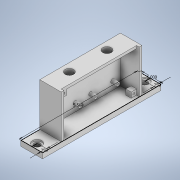
# Autodesk Inventor part: DualSensorReadout
Saved by Autodesk Inventor 2020 (Build 240168000, 168)
## iProperties
Created: 2024-01-28
Part Number: DualSensorReadout
Material: Generic
Document SubType Name: Modeling
Designer: Beaucage
Density: 1 g/cm^3
Appearance: Default
Author: Beaucage
Autodesk Inventor part; units mm, degrees
ref_plane "YZ Plane" through (0, 0, 0) normal (1, 0, 0) x (0, 1, 0)
ref_plane "XZ Plane" through (0, 0, 0) normal (0, 1, 0) x (-1, 0, 0)
ref_plane "XY Plane" through (0, 0, 0) normal (0, 0, 1) x (1, 0, 0)
sketch "Sketch1" plane through (0, 0, 0) normal (0, 1, 0) x (-1, 0, 0)
  line L0 (0, 0) -> (25.4, 0)
  line L1 (25.4, 0) -> (25.4, -139.7)
  line L2 (25.4, -139.7) -> (0, -139.7)
  line L3 (0, -139.7) -> (0, 0)
  line L4 (12.7, 0) -> (12.7, -6.35)
  line L5 (12.7, -139.7) -> (12.7, -133.35)
  dimension "d0" = 25.4
  dimension "d1" = 139.7
  dimension "d2" = 6.35
  dimension "d3" = 6.35
  constraints: 12 end point, 2 midpoint, 2 parallel, 2 vertical, 1 horizontal, 1 perpendicular
  measures "d0" distance of L1.end L2.end
  measures "d1" distance of L0.end L1.end
  measures "d2" distance of L4.start L4.end
  measures "d3" distance of L5.start L5.end
extrude "Extrusion1" add sketch "Sketch1" against normal blind 6.35
hole "Hole1" at (-12.7, 0, -6.35) at (-12.7, 0, -133.35) direction (0, -1, 0) diameter 7.1374 depth 7.9375 counterbore diameter 11.1252 counterbore depth 1.5875 clearance for "Socket Head Cap Screw" size "1/4" standard "Ansi Unified Screw Threads"
sketch "Sketch2" plane through (0, 0, 0) normal (0, 1, 0) x (1, 0, 0)
  line L0 (-25.4, 0) -> (-25.4, 139.7) projected
  line L1 (-25.4, 0) -> (-25.4, 25.4)
  line L2 (-25.4, 25.4) -> (-22.225, 25.4)
  line L3 (-22.225, 25.4) -> (-22.225, 114.3)
  line L4 (-22.225, 114.3) -> (-25.4, 114.3)
  line L5 (-25.4, 114.3) -> (-25.4, 25.4)
  line L6 (-25.4, 25.4) -> (0, 25.4)
  line L7 (0, 25.4) -> (0, 22.225)
  line L8 (0, 22.225) -> (-25.4, 22.225)
  line L9 (-25.4, 22.225) -> (-25.4, 25.4)
  line L10 (-25.4, 114.3) -> (0, 114.3)
  line L11 (0, 114.3) -> (0, 117.475)
  line L12 (0, 117.475) -> (-25.4, 117.475)
  line L13 (-25.4, 117.475) -> (-25.4, 114.3)
  point P0 (0, 0)
  dimension "d13" = 25.4
  dimension "d14" = 3.175
  dimension "d15" = 88.9
  dimension "d16" = 25.4
  dimension "d17" = 3.175
  dimension "d18" = 25.4
  dimension "d19" = 3.175
  constraints: 26 end point, 6 parallel, 3 horizontal, 3 perpendicular, 1 point on line
  measures "d13" distance of L0.start L1.end
  measures "d14" distance of L4.end L3.end
  measures "d15" distance of L3.end L2.end
  measures "d16" distance of L7.end L8.end
  measures "d17" distance of L6.end L7.end
  measures "d18" distance of L12.end L11.end
  measures "d19" distance of L11.end L10.end
extrude "Extrusion2" add sketch "Sketch2" along normal blind 50.8
sketch "Sketch3" plane through (-22.225, 0, -25.4) normal (1, 0, 0) x (0, 0, -1)
  line L0 (88.9, 0) -> (88.9, 50.8) projected
  line L1 (88.9, 50.8) -> (0, 50.8)
  line L2 (0, 50.8) -> (0, 47.625)
  line L3 (0, 47.625) -> (88.9, 47.625)
  line L4 (88.9, 47.625) -> (88.9, 50.8)
  point P0 (-25.4, 0)
  dimension "d22" = 88.9
  dimension "d23" = 3.175
  constraints: 8 end point, 2 parallel, 1 horizontal, 1 perpendicular
  measures "d22" distance of L3.end L2.end
  measures "d23" distance of L2.end L1.end
extrude "Extrusion3" add sketch "Sketch3" along normal blind 19.05
sketch "Sketch4" plane through (-22.225, 0, -25.4) normal (1, 0, 0) x (0, 0, -1)
  line L0 (88.9, 47.625) -> (0, 47.625) projected
  line L1 (44.45, 47.625) -> (44.45, 23.8125)
  line L2 (44.45, 23.8125) -> (66.675, 23.8125)
  line L3 (66.675, 23.8125) -> (22.225, 23.8125)
  line L4 (9.2075, 9.525) -> (35.2425, 9.525)
  line L5 (35.2425, 9.525) -> (35.2425, 38.1)
  line L6 (35.2425, 38.1) -> (9.2075, 38.1)
  line L7 (9.2075, 38.1) -> (9.2075, 9.525)
  line L8 (9.2075, 9.525) -> (35.2425, 38.1) construction
  line L9 (35.2425, 9.525) -> (9.2075, 38.1) construction
  line L10 (53.6575, 9.525) -> (79.6925, 9.525)
  line L11 (79.6925, 9.525) -> (79.6925, 38.1)
  line L12 (79.6925, 38.1) -> (53.6575, 38.1)
  line L13 (53.6575, 38.1) -> (53.6575, 9.525)
  line L14 (53.6575, 9.525) -> (79.6925, 38.1) construction
  line L15 (79.6925, 9.525) -> (53.6575, 38.1) construction
  circle A0 centre (9.2075, 38.1) radius 2.2225
  circle A1 centre (35.2425, 38.1) radius 2.2225
  circle A2 centre (9.2075, 9.525) radius 2.2225
  circle A3 centre (35.2425, 9.525) radius 2.2225
  circle A4 centre (53.6575, 9.525) radius 2.2225
  circle A5 centre (79.6925, 9.525) radius 2.2225
  circle A6 centre (79.6925, 38.1) radius 2.2225
  circle A7 centre (53.6575, 38.1) radius 2.2225
  line L16 (6.6675, 6.985) -> (37.7825, 6.985)
  line L17 (37.7825, 6.985) -> (37.7825, 40.64)
  line L18 (37.7825, 40.64) -> (6.6675, 40.64)
  line L19 (6.6675, 40.64) -> (6.6675, 6.985)
  line L20 (6.6675, 6.985) -> (37.7825, 40.64) construction
  line L21 (37.7825, 6.985) -> (6.6675, 40.64) construction
  line L22 (51.1175, 6.985) -> (82.2325, 6.985)
  line L23 (82.2325, 6.985) -> (82.2325, 40.64)
  line L24 (82.2325, 40.64) -> (51.1175, 40.64)
  line L25 (51.1175, 40.64) -> (51.1175, 6.985)
  line L26 (51.1175, 6.985) -> (82.2325, 40.64) construction
  line L27 (82.2325, 6.985) -> (51.1175, 40.64) construction
  point P0 (-25.4, 0)
  dimension "d26" = 23.8125
  dimension "d27" = 22.225
  dimension "d28" = 44.45
  dimension "d29" = 26.035
  dimension "d30" = 28.575
  dimension "d31" = 26.035
  dimension "d32" = 28.575
  dimension "d33" = 4.445
  dimension "d34" = 4.445
  dimension "d35" = 4.445
  dimension "d36" = 4.445
  dimension "d37" = 4.445
  dimension "d38" = 4.445
  dimension "d39" = 4.445
  dimension "d49" = 31.115
  dimension "d50" = 33.655
  dimension "d51" = 31.115
  dimension "d52" = 33.655
  constraints: 54 end point, 9 midpoint, 8 centre point, 8 coincident, 8 parallel, 5 perpendicular, 4 horizontal, 1 point on line, 1 vertical
  measures "d26" distance of L1.start L1.end
  measures "d27" distance of L1.end L2.end
  measures "d28" distance of L2.end L3.end
  measures "d29" distance of L6.end L5.end
  measures "d30" distance of L5.end L4.end
  measures "d31" distance of L12.end L11.end
  measures "d32" distance of L11.end L10.end
  measures "d33" diameter of A0
  measures "d34" diameter of A1
  measures "d35" diameter of A2
  measures "d36" diameter of A3
  measures "d37" diameter of A4
  measures "d38" diameter of A5
  measures "d39" diameter of A7
  measures "d49" distance of L18.end L17.end
  measures "d50" distance of L17.end L16.end
  measures "d51" distance of L24.end L23.end
  measures "d52" distance of L23.end L22.end
extrude "Extrusion4" add sketch "Sketch4" along normal blind 6.35 contours L7 A2 L4 | L4 A2 L7 | A3 L5 L4 | L4 L5 A3 | A0 L6 L7 | L7 L6 A0 | A1 L5 L6 | L6 L5 A1 | L13 A4 L10 | L10 A4 L13 | A5 L11 L10 | L10 L11 A5 | A7 L12 L13 | L13 L12 A7 | A6 L12 L11 | L11 L12 A6
sketch "Sketch5" plane through (-15.875, 38.1, -34.6075) normal (1, 0, 0) x (0, 0, -1)
  circle A0 centre (0, 0) radius 2.2225 projected
  circle A1 centre (0, -28.575) radius 2.2225 projected
  circle A2 centre (26.035, -28.575) radius 2.2225 projected
  circle A3 centre (26.035, 0) radius 2.2225 projected
  circle A4 centre (44.45, 0) radius 2.2225 projected
  circle A5 centre (70.485, 0) radius 2.2225 projected
  circle A6 centre (70.485, -28.575) radius 2.2225 projected
  circle A7 centre (44.45, -28.575) radius 2.2225 projected
  point P0 (-34.6075, -38.1)
hole "Hole2" at (-15.875, 38.1, -34.6075) at (-15.875, 9.525, -34.6075) at (-15.875, 38.1, -60.6425) at (-15.875, 9.525, -60.6425) at (-15.875, 9.525, -79.0575) at (-15.875, 38.1, -79.0575) at (-15.875, 38.1, -105.0925) at (-15.875, 9.525, -105.0925) direction (-1, 0, 0) diameter 1.778 depth 9.525
sketch "Sketch6" plane through (0, 50.8, 0) normal (0, 1, 0) x (1, 0, 0)
  line L0 (-22.225, 36.83) -> (-22.225, 32.385) projected
  line L1 (-15.875, 32.385) -> (-15.875, 36.83) projected
  line L2 (-15.875, 58.42) -> (-15.875, 62.865) projected
  line L3 (-15.875, 76.835) -> (-15.875, 81.28) projected
  line L4 (-15.875, 102.87) -> (-15.875, 107.315) projected
  line L5 (-22.225, 62.865) -> (-22.225, 58.42) projected
  line L6 (-22.225, 107.315) -> (-22.225, 102.87) projected
  line L7 (-22.225, 81.28) -> (-22.225, 76.835) projected
  line L8 (-22.225, 62.865) -> (-22.225, 58.42) projected
  line L9 (-22.225, 36.83) -> (-22.225, 32.385) projected
  line L10 (-22.225, 107.315) -> (-22.225, 102.87) projected
  line L11 (-22.225, 81.28) -> (-22.225, 76.835) projected
  line L12 (-22.225, 36.83) -> (-22.225, 32.385) projected
  line L13 (-22.225, 114.3) -> (-22.225, 25.4) projected
  line L14 (-22.225, 114.3) -> (-22.225, 25.4) projected
  line L15 (-15.875, 32.385) -> (-15.875, 36.83) projected
  line L16 (-15.875, 36.83) -> (-15.875, 47.625)
  line L17 (-15.875, 76.835) -> (-15.875, 81.28) projected
  line L18 (-15.875, 81.28) -> (-15.875, 92.075)
  point P0 (0, 0)
  dimension "d53" = 10.795
  dimension "d54" = 10.795
  constraints: 4 end point, 2 vertical
  measures "d53" distance of L1.end L16.end
  measures "d54" distance of L3.end L18.end
hole "Hole3" at (-15.875, 50.8, -47.625) at (-15.875, 50.8, -92.075) direction (0, -1, 0) diameter 10.16 depth 9.525
sketch "Sketch8" plane through (-22.225, 47.625, -114.3) normal (0, -1, 0) x (1, 0, 0)
  circle A0 centre (6.35, 66.675) radius 5.08 projected
  line L0 (6.35, 61.595) -> (6.35, 58.42)
  circle A1 centre (6.35, 66.675) radius 5.08 projected
  line L1 (6.35, 71.755) -> (6.35, 74.93)
  circle A2 centre (6.35, 22.225) radius 5.08 projected
  line L2 (6.35, 27.305) -> (6.35, 30.48)
  line L3 (6.35, 17.145) -> (6.35, 13.97)
  arc A3 (6.35, 74.93) -> (6.35, 58.42) centre (6.1206, 66.675) ccw
  arc A4 (6.35, 30.48) -> (6.35, 13.97) centre (6.35, 22.225) ccw
  point P0 (22.225, 114.3)
  point P1 (6.35, 71.755)
  dimension "d66" = 3.175
  dimension "d67" = 3.175
  dimension "d68" = 3.175
  dimension "d69" = 3.175
  dimension "d70" = 8.255
  constraints: 8 end point, 7 point on circle, 4 vertical, 2 centre point, 2 other
  measures "d66" distance of L0.start L0.end
  measures "d67" distance of L1.start L1.end
  measures "d68" distance of L2.start L2.end
  measures "d69" distance of L3.start L3.end
  measures "d70" radius of A4
extrude "Extrusion6" add sketch "Sketch8" along normal blind 6.35 contours A0 L0 A3 L1 | A2 L3 A4 L2
sketch "Sketch9" plane through (-22.225, 0, -25.4) normal (1, 0, 0) x (0, 0, -1)
  line L0 (27.305, 41.275) -> (17.145, 41.275) projected
  line L1 (0, 47.625) -> (88.9, 47.625) projected
  line L2 (17.145, 41.275) -> (10.795, 41.275)
  line L3 (10.795, 41.275) -> (10.795, 47.625)
  line L4 (10.795, 47.625) -> (17.145, 47.625)
  line L5 (17.145, 47.625) -> (17.145, 41.275)
  line L6 (27.305, 47.625) -> (27.305, 41.275) projected
  line L7 (27.305, 41.275) -> (33.655, 41.275)
  line L8 (33.655, 41.275) -> (33.655, 47.625)
  line L9 (33.655, 47.625) -> (27.305, 47.625)
  line L10 (27.305, 47.625) -> (27.305, 41.275)
  line L11 (58.42, 41.275) -> (61.4003, 41.275) projected
  line L12 (61.4003, 41.275) -> (55.0503, 41.275)
  line L13 (55.0503, 41.275) -> (55.0503, 47.625)
  line L14 (55.0503, 47.625) -> (61.4003, 47.625)
  line L15 (61.4003, 47.625) -> (61.4003, 41.275)
  line L16 (74.93, 41.275) -> (71.755, 41.275) projected
  line L17 (71.755, 41.275) -> (78.105, 41.275)
  line L18 (78.105, 41.275) -> (78.105, 47.625)
  line L19 (78.105, 47.625) -> (71.755, 47.625)
  line L20 (71.755, 47.625) -> (71.755, 41.275)
  point P0 (-25.4, 0)
  point P1 (71.755, 47.625)
  point P2 (78.105, 47.625)
  point P3 (61.4003, 47.625)
  point P4 (55.0503, 47.625)
  dimension "d73" = 6.35
  dimension "d74" = 6.35
  dimension "d75" = 6.35
  dimension "d76" = 6.35
  dimension "d77" = 6.35
  constraints: 32 end point, 8 parallel, 4 horizontal, 4 perpendicular, 3 point on line
  measures "d73" distance of L3.end L4.end
  measures "d74" distance of L9.end L8.end
  measures "d75" distance of L13.end L14.end
  measures "d76" distance of L12.end L13.end
  measures "d77" distance of L19.end L18.end
extrude "Extrusion7" add sketch "Sketch9" along normal blind 6.35 contours L6 L1 L8 L7 | L2 L3 L1 L5 | L1 L15 L11 L12 L13 | L1 L18 L17 L16 L20
sketch "Sketch10" plane through (-3.175, 0, -25.4) normal (1, 0, 0) x (0, 0, -1)
  line L0 (0, 47.625) -> (88.9, 47.625) projected
  line L1 (0, 47.625) -> (6.35, 47.625)
  line L2 (6.35, 47.625) -> (6.35, 41.275)
  line L3 (6.35, 41.275) -> (0, 41.275)
  line L4 (0, 41.275) -> (0, 47.625)
  line L5 (88.9, 0) -> (82.55, 0)
  line L6 (82.55, 0) -> (82.55, 6.35)
  line L7 (82.55, 6.35) -> (88.9, 6.35)
  line L8 (88.9, 6.35) -> (88.9, 0)
  point P0 (-25.4, 0)
  point P1 (6.35, 47.625)
  dimension "d80" = 6.35
  dimension "d81" = 6.35
  dimension "d82" = 6.35
  dimension "d83" = 6.35
  constraints: 16 end point, 4 parallel, 2 horizontal, 2 perpendicular
  measures "d80" distance of L2.end L3.end
  measures "d81" distance of L1.end L2.end
  measures "d82" distance of L6.end L7.end
  measures "d83" distance of L5.end L6.end
extrude "Extrusion8" add sketch "Sketch10" against normal blind 6.35
sketch "Sketch11" plane through (-3.175, 0, -25.4) normal (1, 0, 0) x (0, 0, -1)
  line L0 (6.35, 47.625) -> (6.35, 41.275) projected
  line L1 (6.35, 41.275) -> (3.175, 41.275)
  line L2 (3.175, 41.275) -> (3.175, 44.45)
  line L3 (3.175, 44.45) -> (6.35, 44.45)
  line L4 (6.35, 44.45) -> (6.35, 41.275)
  line L5 (82.55, 0) -> (82.55, 6.35) projected
  line L6 (82.55, 6.35) -> (85.725, 6.35)
  line L7 (85.725, 6.35) -> (85.725, 3.175)
  line L8 (85.725, 3.175) -> (82.55, 3.175)
  line L9 (82.55, 3.175) -> (82.55, 6.35)
  point P0 (-25.4, 0)
  dimension "d86" = 3.175
  dimension "d87" = 3.175
  dimension "d88" = 3.175
  constraints: 16 end point, 4 parallel, 2 horizontal, 2 perpendicular
  measures "d86" distance of L2.end L3.end
  measures "d87" distance of L7.end L8.end
  measures "d88" distance of L6.end L7.end
hole "Hole4" at (-3.175, 44.45, -28.575) at (-3.175, 3.175, -111.125) direction (-1, 0, 0) diameter 2.2606 depth 9.525
sketch "Sketch12" plane through (-15.875, 41.275, -42.545) normal (1, 0, 0) x (0, 0, -1)
  line L0 (-6.35, 6.35) -> (-6.35, 0) projected
  line L1 (-6.35, 0) -> (-3.175, 0)
  line L2 (-3.175, 0) -> (-3.175, 3.175)
  line L3 (-3.175, 3.175) -> (-6.35, 3.175)
  line L4 (-6.35, 3.175) -> (-6.35, 0)
  line L5 (10.3523, 0) -> (13.5273, 0)
  line L6 (13.5273, 0) -> (13.5273, 3.175)
  line L7 (13.5273, 3.175) -> (10.3523, 3.175)
  line L8 (10.3523, 3.175) -> (10.3523, 0)
  line L9 (60.96, 0) -> (37.9053, 0) projected
  line L10 (37.9053, 0) -> (41.0803, 0)
  line L11 (41.0803, 0) -> (41.0803, 3.175)
  line L12 (41.0803, 3.175) -> (37.9053, 3.175)
  line L13 (37.9053, 3.175) -> (37.9053, 0)
  line L14 (54.61, 0) -> (60.96, 0) projected
  line L15 (60.96, 0) -> (57.785, 0)
  line L16 (57.785, 0) -> (57.785, 3.175)
  line L17 (57.785, 3.175) -> (60.96, 3.175)
  line L18 (60.96, 3.175) -> (60.96, 0)
  point P0 (-42.545, -41.275)
  dimension "d96" = 3.175
  dimension "d97" = 3.175
  dimension "d98" = 3.175
  dimension "d99" = 3.175
  dimension "d100" = 3.175
  dimension "d101" = 3.175
  dimension "d102" = 3.175
  constraints: 32 end point, 8 parallel, 4 horizontal, 4 perpendicular, 2 point on line
  measures "d96" distance of L3.end L2.end
  measures "d97" distance of L2.end L1.end
  measures "d98" distance of L7.end L6.end
  measures "d99" distance of L12.end L11.end
  measures "d100" distance of L11.end L10.end
  measures "d101" distance of L16.end L17.end
  measures "d102" distance of L15.end L16.end
hole "Hole5" at (-15.875, 44.45, -39.37) at (-15.875, 44.45, -56.0723) at (-15.875, 44.45, -83.6253) at (-15.875, 44.45, -100.33) direction (-1, 0, 0) diameter 2.2606 depth 6.35
body "Solid1"
